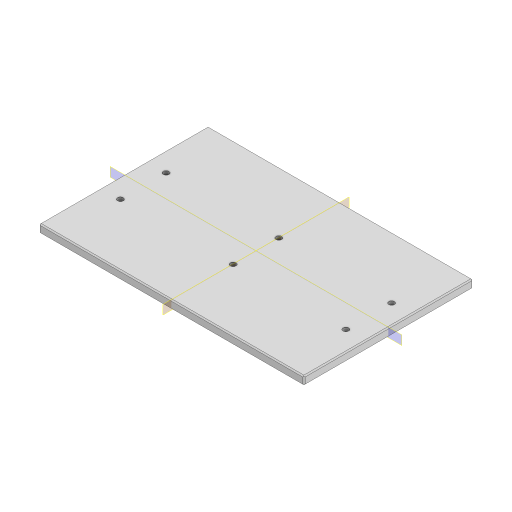
# Autodesk Inventor part: Bodenplatte-Segment
Saved by Autodesk Inventor 2024.3 (Build 283343000, 343)
## iProperties
Created: 2025-05-14
Part Number: Bodenplatte-Segment
Material: Generisch
Document SubType Name: Modeling
Designer: Demir
Density: 1 g/cm^3
Appearance: Vorgabe
Author: Demir
Autodesk Inventor part; units mm, degrees
ref_plane "XY Plane" through (0, 0, 0) normal (0, 0, 1) x (1, 0, 0)
sketch "Skizze1" plane through (0, 0, 0) normal (0, 0, 1) x (1, 0, 0)
  line L0 (-235, 150) -> (235, 150)
  line L1 (235, 150) -> (235, -150)
  line L2 (235, -150) -> (-235, -150)
  line L3 (-235, -150) -> (-235, 150)
  line L4 (-235, 150) -> (235, -150) construction
  line L5 (235, 150) -> (-235, -150) construction
  point P0 (0, 0)
  dimension "d0" = 300
  dimension "d1" = 470
  constraints: 12 end point, 2 midpoint, 2 parallel, 1 horizontal, 1 perpendicular
  measures "d0" distance of L0.end L1.end
  measures "d1" distance of L0.start L0.end
extrude "Extrusion1" add sketch "Skizze1" against normal blind 15
sketch "Skizze2" plane through (0, 0, -15) normal (0, 0, -1) x (-1, 0, 0)
  line L0 (-235, -150) -> (235, -150) projected
  line L1 (235, -150) -> (235, 150) projected
  line L2 (235, 150) -> (-235, 150) projected
  line L3 (-235, 150) -> (-235, -150) projected
  point P0 (0, 0)
  point P1 (0, 40.5)
  point P2 (0, -40.5)
  dimension "d4" = 40.5
  dimension "d5" = 40.5
  constraints: 2 vertical alignment
  measures "d4" distance of point (0, 0) point (0, 40.5)
  measures "d5" distance of point (0, -40.5) point (0, 0)
hole "Bohrung1" at (0, 40.5, -15) at (0, -40.5, -15) direction (0, 0, 1) diameter 9 end through all counterbore diameter 15 counterbore depth 9
pattern_linear "Rechteckige Anordnung1" count 2 spacing 200 along (1, 0, 0) count 2 spacing 200 along (-1, 0, 0) of "Bohrung1"
chamfer "Fasen1" distance 2 angle 45 4 edges at (235, -150, -7.5) (235, 150, -7.5) (-235, 150, -7.5) (-235, -150, -7.5)
chamfer "Fasen2" distance 2 angle 45 8 edges at (0, -150, -15) (0, -150, 0) (-235, 0, 0) (-235, 0, -15) (0, 150, 0) (0, 150, -15) (235, 0, 0) (235, 0, -15)
chamfer "Fasen3" distance 0.5 angle 45 6 edges at (-200, -48, -15) (-200, 33, -15) (0, -48, -15) (0, 33, -15) (200, -48, -15) (200, 33, -15)
chamfer "Fasen4" distance 0.5 angle 45 6 edges at (-200, -45, 0) (-200, 36, 0) (0, -45, 0) (0, 36, 0) (200, -45, 0) (200, 36, 0)
